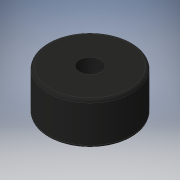
# Autodesk Inventor part: Bumper
Saved by Autodesk Inventor 2017 (Build 210142000, 142)
## iProperties
Created: 2017-05-01
Part Number: Bumper
Material: Generic
Document SubType Name: Modeling
Designer: jeffkub
Density: 1 g/cm^3
Appearance: Default(1)
Author: jeffkub
Autodesk Inventor part; units mm, degrees
ref_plane "YZ Plane" through (0, 0, 0) normal (1, 0, 0) x (0, 1, 0)
ref_plane "XZ Plane" through (0, 0, 0) normal (0, 1, 0) x (-1, 0, 0)
ref_plane "XY Plane" through (0, 0, 0) normal (0, 0, 1) x (1, 0, 0)
sketch "Sketch1" plane through (0, 0, 0) normal (0, 1, 0) x (-1, 0, 0)
  circle A0 centre (0, 0) radius 6.35
  circle A1 centre (0, 0) radius 1.5875
  circle A2 centre (0, 0) radius 3.175
  dimension "d0" = 12.7
  dimension "d1" = 3.175
  dimension "d4" = 6.35
  constraints: 3 centre point, 3 coincident
  measures "d0" diameter of A0
  measures "d1" diameter of A1
  measures "d4" diameter of A2
extrude "Extrusion1" add sketch "Sketch1" along normal blind 6.35 contours A0 | A2
extrude "Extrusion2" cut sketch "Sketch1" along normal blind 3.175 contours A1 | A2
fillet "Fillet1" radius 0.4 2 edges at (6.35, 6.35, 0) (6.35, 0, 0)
body "Solid1"
